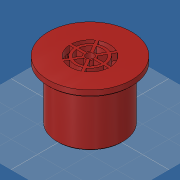
# Autodesk Inventor part: Unterdruckventil_Basis
Saved by Autodesk Inventor 2019 (Build 230136000, 136)
## iProperties
Created: 2020-09-01
Part Number: Unterdruckventil_Basis
Material: Generisch
Document SubType Name: Modeling
Designer: Stefan
Mass: 34.6842 g
Surface Area: 210.694 cm^2
Volume: 34.6842 cm^3
Density: 1 g/cm^3
Appearance: Orangerot
Author: Stefan
Autodesk Inventor part; units mm, degrees
ref_plane "YZ Plane" through (0, 0, 0) normal (1, 0, 0) x (0, 1, 0)
ref_plane "XZ Plane" through (0, 0, 0) normal (0, 1, 0) x (-1, 0, 0)
ref_plane "XY Plane" through (0, 0, 0) normal (0, 0, 1) x (1, 0, 0)
sketch "Skizze1" plane through (0, 0, 0) normal (0, 0, 1) x (1, 0, 0)
  line L0 (-25, -40) -> (-25, 0)
  line L1 (-25, 0) -> (-31.75, 0)
  line L2 (-31.75, 0) -> (-31.75, 5)
  line L3 (-31.75, 5) -> (-15, 5)
  line L4 (-22, -40) -> (-22, -4.0415)
  line L5 (-22, -4.0415) -> (-15, 0)
  line L6 (-15, 0) -> (-15, 5)
  line L7 (-38.1, 0) -> (6.35, 0) construction
  line L8 (-22, -40) -> (-25, -40)
  line L9 (0, -49) -> (0, 14) projected
  point P0 (0, 0)
  dimension "d2" = 60
  dimension "d3" = 3
  dimension "d4" = 5
  dimension "d5" = 7
  dimension "d6" = 50
  dimension "d7" = 40
  dimension "d8" = 63.5
  dimension "d38" = 5
  dimension "d47" = 30
  constraints: 16 end point, 5 perpendicular, 1 collinear, 1 vertical
  measures "d2" angle of L4 L5
  measures "d3" distance between parallel lines of L4 L0
  measures "d4" distance between parallel lines of L1 L3
  measures "d5" distance between parallel lines of L6 L4
  measures "d6" diameter of L0 L9
  measures "d7" distance between parallel lines of L8 L1
  measures "d8" diameter of L2 L9
  measures "d38" distance from line of L5.end L3
  measures "d47" diameter of L6 L9
revolve "Umdrehung1" add sketch "Skizze1" angle 360 about axis through (0, -10, 0) along (0, 1, 0)
sketch "Skizze2" plane through (0, 5, 0) normal (0, 1, 0) x (1, 0, 0)
  circle A0 centre (0, 0) radius 15 projected
  circle A1 centre (0, 0) radius 31.75 projected
  line L0 (-44.45, 0) -> (44.45, 0) construction
  line L1 (0, 44.45) -> (0, -44.45) construction
  circle A2 centre (0, 0) radius 9.5
  circle A3 centre (0, 0) radius 11.5
  circle A4 centre (0, 0) radius 4
  circle A5 centre (0, 0) radius 3
  line L2 (-14.9666, 1) -> (-3.873, 1)
  line L3 (-3.873, -1) -> (-14.9666, -1)
  arc A6 (-3.873, 1) -> (-3.873, -1) centre (0, 0) ccw
  arc A7 (-14.9666, 1) -> (-14.9666, -1) centre (0, 0) ccw
  line L4 (-8.3493, -12.4615) -> (-2.8025, -2.8541)
  line L5 (-1.0705, -3.8541) -> (-6.6173, -13.4615)
  arc A8 (-8.3493, -12.4615) -> (-6.6173, -13.4615) centre (0, 0) ccw
  arc A9 (-2.8025, -2.8541) -> (-1.0705, -3.8541) centre (0, 0) ccw
  line L6 (6.6173, -13.4615) -> (1.0705, -3.8541)
  line L7 (2.8025, -2.8541) -> (8.3493, -12.4615)
  arc A10 (6.6173, -13.4615) -> (8.3493, -12.4615) centre (0, 0) ccw
  arc A11 (1.0705, -3.8541) -> (2.8025, -2.8541) centre (0, 0) ccw
  line L8 (14.9666, -1) -> (3.873, -1)
  line L9 (3.873, 1) -> (14.9666, 1)
  arc A12 (14.9666, -1) -> (14.9666, 1) centre (0, 0) ccw
  arc A13 (3.873, -1) -> (3.873, 1) centre (0, 0) ccw
  line L10 (8.3493, 12.4615) -> (2.8025, 2.8541)
  line L11 (1.0705, 3.8541) -> (6.6173, 13.4615)
  arc A14 (8.3493, 12.4615) -> (6.6173, 13.4615) centre (0, 0) ccw
  arc A15 (2.8025, 2.8541) -> (1.0705, 3.8541) centre (0, 0) ccw
  line L12 (-6.6173, 13.4615) -> (-1.0705, 3.8541)
  line L13 (-2.8025, 2.8541) -> (-8.3493, 12.4615)
  arc A16 (-6.6173, 13.4615) -> (-8.3493, 12.4615) centre (0, 0) ccw
  arc A17 (-1.0705, 3.8541) -> (-2.8025, 2.8541) centre (0, 0) ccw
  dimension "d25" = 19
  dimension "d26" = 23
  dimension "d28" = 8
  dimension "d29" = 6
  dimension "d30" = 2
  dimension "d41" = 360
  constraints: 26 point on circle, 24 end point, 16 centre point, 4 coincident, 3 concentric, 1 horizontal, 1 parallel, 62 other
  measures "d25" diameter of A2
  measures "d26" diameter of A3
  measures "d28" diameter of A4
  measures "d29" diameter of A5
  measures "d30" distance between parallel lines of L3 L2
extrude "Extrusion1" add sketch "Skizze2" against normal blind 5 contours A0 L8 A3 L9 | L10 A3 L11 A0 | L9 A2 L10 A3 | A3 L8 A2 L9 | A0 L6 A3 L7 | A3 L7 A2 L8 | L10 A2 L11 A3 | A2 L8 A4 L9 | A3 L6 A2 L7 | L12 A3 L13 A0 | L11 A2 L12 A3 | L10 A4 L11 A2 | A4 | A0 L4 A3 L5 | A3 L5 A2 L6 | A2 L6 A4 L7 | L12 A2 L13 A3 | A3 L4 A2 L5 | L2 A3 L3 A0 | L13 A2 L2 A3 | L12 A4 L13 A2 | A3 L3 A2 L4 | A2 L4 A4 L5 | L2 A2 L3 A3 | L2 A4 L3 A2
chamfer "Fase1" distance 1 angle 45 2 edges at (31.75, 0, 0) (25, -40, 0)
sketch "Skizze3" plane through (0, 0, 0) normal (0, -1, 0) x (1, 0, 0)
  circle A0 centre (0, 0) radius 22 projected
  arc A1 (-6.6173, -13.4615) -> (6.6173, -13.4615) centre (0, 0) ccw projected
  line L0 (6.6173, -13.4615) -> (4.8622, -10.4216) projected
  arc A2 (-4.8622, -10.4216) -> (4.8622, -10.4216) centre (0, 0) ccw projected
  line L1 (-4.8622, -10.4216) -> (-6.6173, -13.4615) projected
  line L2 (-8.3493, -12.4615) -> (-6.5942, -9.4216) projected
  arc A3 (-11.4564, -1) -> (-6.5942, -9.4216) centre (0, 0) ccw projected
  line L3 (-11.4564, -1) -> (-14.9666, -1) projected
  arc A4 (-14.9666, -1) -> (-8.3493, -12.4615) centre (0, 0) ccw projected
  line L4 (-14.9666, 1) -> (-11.4564, 1) projected
  arc A5 (-6.5942, 9.4216) -> (-11.4564, 1) centre (0, 0) ccw projected
  line L5 (-6.5942, 9.4216) -> (-8.3493, 12.4615) projected
  arc A6 (-8.3493, 12.4615) -> (-14.9666, 1) centre (0, 0) ccw projected
  line L6 (-6.6173, 13.4615) -> (-4.8622, 10.4216) projected
  arc A7 (4.8622, 10.4216) -> (-4.8622, 10.4216) centre (0, 0) ccw projected
  line L7 (4.8622, 10.4216) -> (6.6173, 13.4615) projected
  arc A8 (6.6173, 13.4615) -> (-6.6173, 13.4615) centre (0, 0) ccw projected
  line L8 (8.3493, 12.4615) -> (6.5942, 9.4216) projected
  arc A9 (11.4564, 1) -> (6.5942, 9.4216) centre (0, 0) ccw projected
  line L9 (11.4564, 1) -> (14.9666, 1) projected
  arc A10 (14.9666, 1) -> (8.3493, 12.4615) centre (0, 0) ccw projected
  arc A11 (3.8576, 8.6815) -> (-3.8576, 8.6815) centre (0, 0) ccw projected
  line L10 (-3.8576, 8.6815) -> (-1.0705, 3.8541) projected
  arc A12 (1.0705, 3.8541) -> (-1.0705, 3.8541) centre (0, 0) ccw projected
  line L11 (1.0705, 3.8541) -> (3.8576, 8.6815) projected
  line L12 (9.4472, -1) -> (3.873, -1) projected
  arc A13 (2.8025, -2.8541) -> (3.873, -1) centre (0, 0) ccw projected
  line L13 (2.8025, -2.8541) -> (5.5896, -7.6815) projected
  arc A14 (5.5896, -7.6815) -> (9.4472, -1) centre (0, 0) ccw projected
  circle A15 centre (0, 0) radius 3 projected
  line L14 (3.8576, -8.6815) -> (1.0705, -3.8541) projected
  arc A16 (-1.0705, -3.8541) -> (1.0705, -3.8541) centre (0, 0) ccw projected
  line L15 (-1.0705, -3.8541) -> (-3.8576, -8.6815) projected
  arc A17 (-3.8576, -8.6815) -> (3.8576, -8.6815) centre (0, 0) ccw projected
  line L16 (5.5896, 7.6815) -> (2.8025, 2.8541) projected
  arc A18 (3.873, 1) -> (2.8025, 2.8541) centre (0, 0) ccw projected
  line L17 (3.873, 1) -> (9.4472, 1) projected
  arc A19 (9.4472, 1) -> (5.5896, 7.6815) centre (0, 0) ccw projected
  arc A20 (-5.5896, 7.6815) -> (-9.4472, 1) centre (0, 0) ccw projected
  line L18 (-9.4472, 1) -> (-3.873, 1) projected
  arc A21 (-2.8025, 2.8541) -> (-3.873, 1) centre (0, 0) ccw projected
  line L19 (-2.8025, 2.8541) -> (-5.5896, 7.6815) projected
  arc A22 (-9.4472, -1) -> (-5.5896, -7.6815) centre (0, 0) ccw projected
  line L20 (-5.5896, -7.6815) -> (-2.8025, -2.8541) projected
  arc A23 (-3.873, -1) -> (-2.8025, -2.8541) centre (0, 0) ccw projected
  line L21 (-3.873, -1) -> (-9.4472, -1) projected
  line L22 (14.9666, -1) -> (11.4564, -1) projected
  arc A24 (6.5942, -9.4216) -> (11.4564, -1) centre (0, 0) ccw projected
  line L23 (6.5942, -9.4216) -> (8.3493, -12.4615) projected
  arc A25 (8.3493, -12.4615) -> (14.9666, -1) centre (0, 0) ccw projected
  circle A26 centre (0, 0) radius 31.75 projected
  line L24 (21.9773, -1) -> (17.9722, -1)
  line L25 (21.9773, 1) -> (17.9722, 1)
  arc A27 (17.9722, -1) -> (17.9722, 1) centre (0, 0) ccw
  arc A28 (21.9773, -1) -> (21.9773, 1) centre (0, 0) ccw
  arc A29 (9.8521, 15.0644) -> (8.1201, 16.0644) centre (0, 0) ccw
  line L26 (11.8547, 18.5329) -> (9.8521, 15.0644)
  arc A30 (11.8547, 18.5329) -> (10.1226, 19.5329) centre (0, 0) ccw
  line L27 (10.1226, 19.5329) -> (8.1201, 16.0644)
  arc A31 (-8.1201, 16.0644) -> (-9.8521, 15.0644) centre (0, 0) ccw
  line L28 (-10.1226, 19.5329) -> (-8.1201, 16.0644)
  arc A32 (-10.1226, 19.5329) -> (-11.8547, 18.5329) centre (0, 0) ccw
  line L29 (-11.8547, 18.5329) -> (-9.8521, 15.0644)
  arc A33 (-17.9722, 1) -> (-17.9722, -1) centre (0, 0) ccw
  line L30 (-21.9773, 1) -> (-17.9722, 1)
  arc A34 (-21.9773, 1) -> (-21.9773, -1) centre (0, 0) ccw
  line L31 (-21.9773, -1) -> (-17.9722, -1)
  arc A35 (-9.8521, -15.0644) -> (-8.1201, -16.0644) centre (0, 0) ccw
  line L32 (-11.8547, -18.5329) -> (-9.8521, -15.0644)
  arc A36 (-11.8547, -18.5329) -> (-10.1226, -19.5329) centre (0, 0) ccw
  line L33 (-10.1226, -19.5329) -> (-8.1201, -16.0644)
  arc A37 (8.1201, -16.0644) -> (9.8521, -15.0644) centre (0, 0) ccw
  line L34 (10.1226, -19.5329) -> (8.1201, -16.0644)
  arc A38 (10.1226, -19.5329) -> (11.8547, -18.5329) centre (0, 0) ccw
  line L35 (11.8547, -18.5329) -> (9.8521, -15.0644)
  dimension "d51" = 18
  dimension "d56" = 360
  constraints: 26 point on circle, 24 end point, 12 centre point, 7 concentric, 2 collinear, 61 other
  measures "d51" radius of A27
extrude "Extrusion5" add sketch "Skizze3" along normal up to surface (40 mm away) contours A0 L24 A27 L25 | L26 A29 L27 A0 | A0 L34 A37 L35 | L28 A31 L29 A0 | A0 L32 A35 L33 | L30 A33 L31 A0
